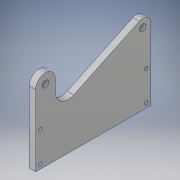
# Autodesk Inventor part: Intake Mount
Saved by Autodesk Inventor 2019.4 (Build 234330000, 330)
## iProperties
Created: 2020-01-06
Part Number: Intake Mount
Material: Aluminum 6061
Document SubType Name: Modeling
Designer: admin
Density: 2.7 g/cm^3
Appearance: Aluminum - Flat
Author: admin
Autodesk Inventor part; units mm, degrees
ref_plane "YZ Plane" through (0, 0, 0) normal (1, 0, 0) x (0, 1, 0)
ref_plane "XZ Plane" through (0, 0, 0) normal (0, 1, 0) x (-1, 0, 0)
ref_plane "XY Plane" through (0, 0, 0) normal (0, 0, 1) x (1, 0, 0)
sketch "Sketch1" plane through (0, 0, 0) normal (1, 0, 0) x (0, 1, 0)
  line L0 (0, 0) -> (0, -177.5)
  circle A0 centre (110, -165) radius 5
  arc A1 (121.3006, -159.6572) -> (110, -177.5) centre (110, -165) ccw construction
  circle A2 centre (110, -15) radius 5
  arc A3 (110, -30) -> (110, 0) centre (110, -15) ccw
  line L1 (0, 0) -> (60, 0)
  line L2 (60, 0) -> (110, 0)
  line L3 (110, -30) -> (60, -30)
  line L4 (60, -30) -> (121.3006, -159.6572)
  line L5 (110, -177.5) -> (0, -177.5)
  line L6 (110, -15) -> (110, -165) construction
  arc A4 (110, 0) -> (110, -30) centre (110, -15) ccw construction
  arc A5 (110, -177.5) -> (121.3006, -159.6572) centre (110, -165) ccw
  line L7 (60, 0) -> (60, -30) construction
  circle A6 centre (7, -7) radius 2.75
  circle A7 centre (53, -7) radius 2.75
  circle A8 centre (53, -170.5) radius 2.75
  circle A9 centre (7, -170.5) radius 2.75
  dimension "d0" = 10
  dimension "d1" = 30
  dimension "d2" = 25
  dimension "d3" = 10
  dimension "d4" = 60
  dimension "d6" = 50
  dimension "d7" = 0
  dimension "d8" = 5.5
  dimension "d9" = 5.5
  dimension "d10" = 5.5
  dimension "d11" = 5.5
  dimension "d12" = 7
  dimension "d13" = 7
  dimension "d14" = 7
  dimension "d15" = 7
  dimension "d16" = 7
  dimension "d17" = 7
  dimension "d18" = 7
  dimension "d19" = 7
  dimension "d23" = 150
  constraints: 16 end point, 10 centre point, 8 point on circle, 4 tangent, 3 vertical, 2 coincident, 1 horizontal, 1 perpendicular, 1 point on line
  measures "d0" diameter of A2
  measures "d1" diameter of A3
  measures "d2" diameter of A1
  measures "d3" diameter of A0
  measures "d4" distance of L0.start L1.end
  measures "d6" distance from line of L1.end L6
  measures "d7" vertical distance of L1.end L2.end
  measures "d8" diameter of A6
  measures "d9" diameter of A7
  measures "d10" diameter of A8
  measures "d11" diameter of A9
  measures "d12" distance from line of L0 A6.centre
  measures "d13" distance from line of L1 A6.centre
  measures "d14" distance from line of L1 A7.centre
  measures "d15" distance from line of L7 A7.centre
  measures "d16" distance from line of L5 A8.centre
  measures "d17" distance from line of L5 A9.centre
  measures "d18" distance from line of L0 A9.centre
  measures "d19" distance from line of L7 A8.centre
  measures "d23" distance of A0.centre A2.centre
extrude "Extrusion1" add sketch "Sketch1" along normal blind 10
fillet "Fillet1" radius 20 1 edges at (5, 60, -30)
body "Solid1"
